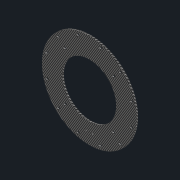
# Autodesk Inventor part: unit-j2-plate1
Saved by Autodesk Inventor 2021 (Build 250183000, 183)
## iProperties
Created: 2021-07-12
Part Number: unit-j2-plate1
Material: CFRP
Document SubType Name: Sheet Metal
Designer: yuta0
Density: 1.43 g/cm^3
Sheet Metal Rule: Default_mm
Appearance: カーボンファイバー
Mass: 22.5141 g
Surface Area: 175.989 cm^2
Volume: 15.7442 cm^3
Author: yuta0
Autodesk Inventor part; units mm, degrees
ref_plane "YZ Plane" through (0, 0, 0) normal (1, 0, 0) x (0, 1, 0)
ref_plane "XZ Plane" through (0, 0, 0) normal (0, 1, 0) x (-1, 0, 0)
ref_plane "XY Plane" through (0, 0, 0) normal (0, 0, 1) x (1, 0, 0)
sketch "スケッチ1" plane through (0, 0, 0) normal (0, 0, 1) x (1, 0, 0)
  circle A0 centre (0, 0) radius 67.5
  dimension "d0" = 135
  measures "d0" diameter of A0
extrude "プレート1" add sketch "スケッチ1" along normal blind 2
sketch "スケッチ2" plane through (0, 0, 2) normal (0, 0, 1) x (1, 0, 0)
  circle A0 centre (0, 0) radius 38.5
  dimension "d2" = 77
  constraints: 1 centre point, 1 coincident
  measures "d2" diameter of A0
extrude "押し出し1" cut sketch "スケッチ2" against normal through all
sketch "スケッチ3" plane through (0, 0, 2) normal (0, 0, 1) x (1, 0, 0)
  circle A0 centre (0, 0) radius 62.5
  point P0 (16.1762, 60.3704)
  point P1 (-16.1762, 60.3704)
  point P2 (-44.1942, 44.1942)
  point P3 (-60.3704, 16.1762)
  point P4 (-60.3704, -16.1762)
  point P5 (-44.1942, -44.1942)
  point P6 (-16.1762, -60.3704)
  point P7 (16.1762, -60.3704)
  point P8 (44.1942, -44.1942)
  point P9 (60.3704, -16.1762)
  point P10 (60.3704, 16.1762)
  point P11 (44.1942, 44.1942)
  dimension "d5" = 125
  dimension "d8" = 360
  dimension "d36" = 0
  constraints: 1 coincident, 16 other
  measures "d36" vertical distance of point (-16.176, 60.37) point (16.176, 60.37)
hole "穴1" at (16.1762, 60.3704, 2) at (-16.1762, 60.3704, 2) at (-44.1942, 44.1942, 2) at (-60.3704, 16.1762, 2) at (-60.3704, -16.1762, 2) at (-44.1942, -44.1942, 2) at (-16.1762, -60.3704, 2) at (16.1762, -60.3704, 2) at (44.1942, -44.1942, 2) at (60.3704, -16.1762, 2) at (60.3704, 16.1762, 2) at (44.1942, 44.1942, 2) direction (0, 0, -1) diameter 4.5 end through all clearance for "Flat Head Machine Screw" size "M4" standard "Ansi Metric M Profile"
sketch "スケッチ4" plane through (0, 0, 2) normal (0, 0, 1) x (1, 0, 0)
  circle A0 centre (0, 0) radius 49
  point P0 (-34.6482, 34.6482)
  point P1 (-34.6482, -34.6482)
  point P2 (34.6482, -34.6482)
  point P3 (34.6482, 34.6482)
  dimension "d17" = 98
  dimension "d20" = 360
  dimension "d29" = 0
  constraints: 1 coincident, 8 other
  measures "d29" vertical distance of point (34.648, 34.648) point (-34.648, 34.648)
hole "穴2" at (-34.6482, 34.6482, 2) at (-34.6482, -34.6482, 2) at (34.6482, -34.6482, 2) at (34.6482, 34.6482, 2) direction (0, 0, -1) diameter 4.5 end through all clearance for "Flat Head Machine Screw" size "M4" standard "Ansi Metric M Profile"
sketch "スケッチ6" plane through (0, 0, 0) normal (0, 0, -1) x (-1, 0, 0)
  circle A0 centre (0, 0) radius 37.5
  line L0 (-4.75, -42.3) -> (4.75, -42.3)
  line L1 (-4.75, -37.5) -> (4.75, -37.5)
  circle A1 centre (0, -37.5) radius 4.8
  point P0 (-4.75, -51.1)
  point P1 (4.75, -51.1)
  dimension "d37" = 75
  dimension "d38" = 9.5
  dimension "d39" = 8.8
  dimension "d40" = 13.6
  dimension "d41" = 4.75
  constraints: 4 end point, 4 vertical alignment, 2 centre point, 2 horizontal, 2 tangent, 1 coincident, 1 horizontal alignment, 1 midpoint
  measures "d37" diameter of A0
  measures "d38" distance of point (-4.75, -51.1) point (4.75, -51.1)
  measures "d39" distance from line of point (4.75, -51.1) L0
  measures "d40" distance from line of point (4.75, -51.1) L1
  measures "d41" horizontal distance of L0.start point (0, 0)
hole "穴3" at (4.75, -51.1, 0) at (-4.75, -51.1, 0) direction (0, 0, 1) diameter 2.4 end through all clearance for "Socket Head Cap Screw" size "M2" standard "Ansi Metric M Profile"
equation "\"d15\" = Thickness"
equation "\"d27\" = Thickness"
equation "\"d47\" = Thickness"
equation "\"d1\" = Thickness"
equation "\"BendRadius\" = Thickness"
equation "\"BendReliefWidth\" = Thickness"
equation "\"BendReliefDepth\" = 0.5 * Thickness"
equation "\"CornerReliefSize\" = 4 * Thickness"
equation "\"MinimumRemnant\" = 2 * Thickness"
equation "\"TransitionRadius\" = BendRadius"
equation "\"JacobiRadiusSize\" = BendRadius"
equation "\"GapSize\" = Thickness"
equation "\"Thickness\" = 2"
